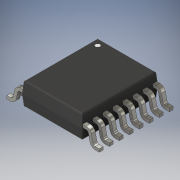
# Autodesk Inventor part: Semiconductor_TSSOP-16
Saved by Autodesk Inventor 2018 (Build 220112000, 112)
## iProperties
Created: 2016-07-22
Part Number: Semiconductor_TSSOP-16
Material: ABS Plastic
Document SubType Name: Modeling
Designer: Bradley
Density: 1.06 g/cm^3
Appearance: Smooth - Black
Mass: 0.00993513 g
Surface Area: 0.40182 cm^2
Volume: 0.00937276 cm^3
Author: Bradley
Autodesk Inventor part; units mm, degrees
ref_plane "YZ Plane" through (0, 0, 0) normal (1, 0, 0) x (0, 1, 0)
ref_plane "XZ Plane" through (0, 0, 0) normal (0, 1, 0) x (-1, 0, 0)
ref_plane "XY Plane" through (0, 0, 0) normal (0, 0, 1) x (1, 0, 0)
sketch "Sketch1" plane through (0, 0, 0) normal (0, 1, 0) x (-1, 0, 0)
  line L0 (-1.95, 2.45) -> (1.95, 2.45)
  line L1 (1.95, 2.45) -> (1.95, -2.45)
  line L2 (1.95, -2.45) -> (-1.95, -2.45)
  line L3 (-1.95, -2.45) -> (-1.95, 2.45)
  line L4 (-1.95, 2.45) -> (1.95, -2.45) construction
  line L5 (1.95, 2.45) -> (-1.95, -2.45) construction
  point P0 (0, 0)
  dimension "d0" = 3.9
  dimension "d1" = 4.9
  constraints: 12 end point, 2 midpoint, 2 parallel, 1 horizontal, 1 perpendicular
  measures "d0" distance of L1.end L2.end
  measures "d1" distance of L0.end L1.end
extrude "Extrusion1" add sketch "Sketch1" along normal blind 0.75 draft -5
sketch "Sketch2" plane through (0, 0, 0) normal (0, -1, 0) x (1, 0, 0)
  line L0 (1.95, 2.45) -> (-1.95, 2.45) projected
  line L1 (1.95, 2.45) -> (-1.95, 2.45) projected
  line L2 (-1.95, 2.45) -> (-1.95, -2.45) projected
  line L3 (-1.95, -2.45) -> (1.95, -2.45) projected
  line L4 (1.95, -2.45) -> (1.95, 2.45) projected
  point P0 (0, 0)
extrude "Extrusion2" add sketch "Sketch2" along normal blind 0.75 draft -5
fillet "Fillet1" radius 0.1 8 edges at (-1.8844, 0.75, 0) (0, 0.75, 2.3844) (0, 0.75, -2.3844) (1.8844, 0.75, 0) (1.8844, -0.75, 0) (0, -0.75, 2.3844) (-1.8844, -0.75, 0) (0, -0.75, -2.3844)
sketch "Sketch3" plane through (0, 0, 0) normal (0, 1, 0) x (-1, 0, 0)
  line L0 (1.95, 2.45) -> (1.95, -2.45) projected
  line L1 (-1.95, 2.45) -> (1.95, 2.45) projected
  line L2 (1.95, 2.4) -> (2.15, 2.4)
  line L3 (2.15, 2.4) -> (2.15, 2.15)
  line L4 (2.15, 2.15) -> (1.95, 2.15)
  line L5 (1.95, 2.15) -> (1.95, 2.4)
  line L6 (-1.95, -2.45) -> (-1.95, 2.45) projected
  line L7 (-1.95, 2.4) -> (-2.15, 2.4)
  line L8 (-2.15, 2.4) -> (-2.15, 2.15)
  line L9 (-2.15, 2.15) -> (-1.95, 2.15)
  line L10 (-1.95, 2.15) -> (-1.95, 2.4)
  line L11 (-1.95, 2.15) -> (1.95, 2.15)
  line L12 (1.95, 2.15) -> (1.95, 2.4)
  line L13 (1.95, 2.4) -> (-1.95, 2.4)
  line L14 (-1.95, 2.4) -> (-1.95, 2.15)
  point P0 (0, 0)
  point P1 (1.95, 2.275)
  dimension "d7" = 0.25
  dimension "d8" = 2.275
  dimension "d9" = 0.2
  constraints: 24 end point, 6 parallel, 4 point on line, 3 horizontal, 3 perpendicular, 1 collinear, 1 midpoint
  measures "d7" distance of L2.end L3.end
  measures "d8" vertical distance of point (1.95, 2.275) point (0, 0)
  measures "d9" distance of L3.end L4.end
extrude "Extrusion3" add sketch "Sketch3" along normal blind 0.2 contours L2 L3 L4 L0 | L0 L11 L6 L13 | L6 L9 L8 L7
sketch "Sketch4" plane through (-2.15, 0, 2.4) normal (0, 0, 1) x (1, 0, 0)
  line L0 (0.2175, 0.2) -> (0.2, 0) projected
  line L1 (0, 0.2) -> (0.2175, 0.2) projected
  line L2 (0, 0) -> (0, 0.2) projected
  line L3 (0, 0) -> (0.2, 0) projected
  line L4 (4.1, 0) -> (4.0825, 0.2) projected
  line L5 (4.1, 0) -> (4.3, 0) projected
  line L6 (4.3, 0) -> (4.3, 0.2) projected
  line L7 (4.0825, 0.2) -> (4.3, 0.2) projected
  line L8 (0, 0) -> (0.2, 0) projected
  arc A0 (0, 0) -> (-0.1463, -0.117) centre (0, -0.15) ccw
  arc A1 (-0.5914, -0.85) -> (-0.25, -0.577) centre (-0.5914, -0.5) ccw
  line L9 (0, 0.2) -> (0.2175, 0.2) projected
  arc A2 (0, 0.2) -> (-0.3414, -0.073) centre (0, -0.15) ccw
  arc A3 (-0.5914, -0.65) -> (-0.4451, -0.533) centre (-0.5914, -0.5) ccw
  line L10 (-0.5914, -0.85) -> (-0.85, -0.85)
  line L11 (-0.85, -0.85) -> (-0.85, -0.65)
  line L12 (-0.85, -0.65) -> (-0.5914, -0.65)
  line L13 (-0.3414, -0.073) -> (-0.4451, -0.533)
  line L14 (-0.1463, -0.117) -> (-0.25, -0.577)
  line L15 (3.9428, -0.75) -> (0.3572, -0.75) projected
  line L16 (0, 0.2) -> (0, 0)
  line L17 (0.3572, 0.75) -> (3.9428, 0.75) projected
  line L18 (2.15, 0.5) -> (2.15, -0.5)
  line L19 (4.3, 0) -> (4.3, 0.2)
  arc A4 (4.4463, -0.117) -> (4.3, 0) centre (4.3, -0.15) ccw
  arc A5 (4.55, -0.577) -> (4.8914, -0.85) centre (4.8914, -0.5) ccw
  arc A6 (4.6414, -0.073) -> (4.3, 0.2) centre (4.3, -0.15) ccw
  arc A7 (4.7451, -0.533) -> (4.8914, -0.65) centre (4.8914, -0.5) ccw
  line L20 (4.8914, -0.85) -> (5.15, -0.85)
  line L21 (5.15, -0.85) -> (5.15, -0.65)
  line L22 (5.15, -0.65) -> (4.8914, -0.65)
  line L23 (4.6414, -0.073) -> (4.7451, -0.533)
  line L24 (4.4463, -0.117) -> (4.55, -0.577)
  point P0 (2.15, 0)
  dimension "d12" = 0.15
  dimension "d13" = 0.15
  dimension "d16" = 0.6
  dimension "d17" = 0.1
  dimension "d25" = 6
  constraints: 26 end point, 16 point on circle, 12 symmetric about line, 8 centre point, 6 tangent, 4 coincident, 2 equal length, 2 perpendicular, 1 horizontal, 1 parallel, 4 other
  measures "d12" radius of A0
  measures "d13" radius of A3
  measures "d16" distance from line of L11 L14.end
  measures "d17" distance between parallel lines of L10 L15
  measures "d25" distance between parallel lines of L21 L11
extrude "Extrusion4" add sketch "Sketch4" against normal up to surface (0.25 mm away) contours L2 A0 L14 A1 L10 L11 L12 A3 L13 A2 | L6 A6 L23 A7 L22 L21 L20 A5 L24 A4
pattern_linear "Rectangular Pattern1" count 8 spacing 0.65 along (0, 0, -1) of "Extrusion4", "Extrusion3"
sketch "Sketch5" plane through (0, 0.75, 0) normal (0, 1, 0) x (1, 0, 0)
  line L0 (1.7928, -2.2928) -> (-1.7928, -2.2928) projected
  line L1 (1.7928, 2.2928) -> (1.7928, -2.2928) projected
  line L2 (-1.7928, 2.2928) -> (1.7928, 2.2928) projected
  line L3 (-1.7928, -2.2928) -> (-1.7928, 2.2928) projected
  circle A0 centre (-1.45, 1.95) radius 0.15
  circle A1 centre (-1.45, 1.95) radius 0.3428 construction
  line L4 (-1.7928, -2.2928) -> (-1.7928, 2.2928) projected
  line L5 (-1.7928, -2.2928) -> (1.7928, -2.2928) construction
  line L6 (-1.7928, 2.2928) -> (1.7928, 2.2928) construction
  line L7 (-1.95, 2.45) -> (1.95, 2.45) projected
  point P0 (0, 0)
  dimension "d26" = 0.5
  dimension "d27" = 0.3
  constraints: 2 centre point, 2 tangent, 1 coincident
  measures "d26" distance from line of A0.centre L7
  measures "d27" diameter of A0
extrude "Extrusion5" add sketch "Sketch5" along normal blind 0.01 and the other way blind 0.255 contours A0
equation "\"d13\" = d12"
body "Solid1"
